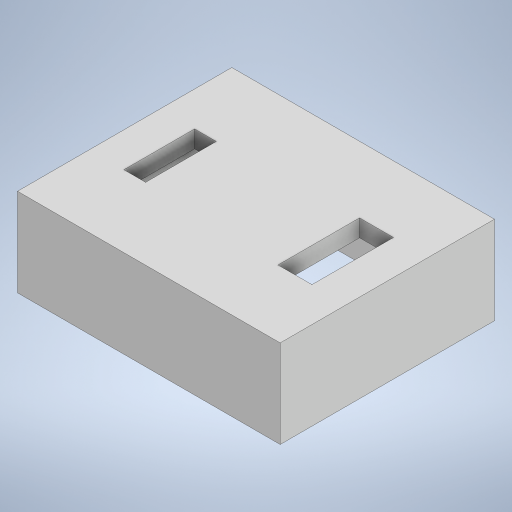
# Autodesk Inventor part: pololuCaseTop
Saved by Autodesk Inventor 2024 (Build 280153000, 153)
## iProperties
Created: 2023-08-07
Part Number: pololuCaseTop
Material: Generic
Document SubType Name: Modeling
Designer: 18179
Density: 1 g/cm^3
Appearance: Default
Author: 18179
Autodesk Inventor part; units mm, degrees
ref_plane "YZ Plane" through (0, 0, 0) normal (1, 0, 0) x (0, 1, 0)
ref_plane "XZ Plane" through (0, 0, 0) normal (0, 1, 0) x (-1, 0, 0)
ref_plane "XY Plane" through (0, 0, 0) normal (0, 0, 1) x (1, 0, 0)
sketch "Sketch1" plane through (0, 0, 0) normal (0, 1, 0) x (-1, 0, 0)
  line L0 (0, 0) -> (41.91, 0)
  line L1 (41.91, 0) -> (41.91, -33.02)
  line L2 (41.91, -33.02) -> (0, -33.02)
  line L3 (0, -33.02) -> (0, 0)
  line L4 (41.91, -16.51) -> (34.735, -16.51)
  line L5 (34.735, -16.51) -> (34.735, -10.01)
  line L6 (34.735, -10.01) -> (41.91, -10.01)
  line L7 (34.735, -10.01) -> (38.735, -10.01)
  line L8 (38.735, -10.01) -> (38.735, -23.01)
  line L9 (38.735, -23.01) -> (34.735, -23.01)
  line L10 (34.735, -23.01) -> (34.735, -10.01)
  line L11 (0, -16.51) -> (9.425, -16.51)
  line L12 (9.425, -16.51) -> (9.425, -9.01)
  line L13 (9.425, -9.01) -> (3.175, -9.01)
  line L14 (3.175, -9.01) -> (3.175, -24.01)
  line L15 (3.175, -24.01) -> (9.425, -24.01)
  line L16 (9.425, -24.01) -> (9.425, -9.01)
  point P0 (0, -9.01)
  point P1 (0, -24.01)
  point P2 (41.91, -23.01)
  point P3 (3.175, -16.51)
  point P4 (38.735, -16.51)
  dimension "d0" = 41.91
  dimension "d1" = 33.02
  dimension "d2" = 7.175
  dimension "d3" = 6.5
  dimension "d4" = 4
  dimension "d5" = 13
  dimension "d6" = 9.425
  dimension "d7" = 7.5
  dimension "d8" = 6.25
  dimension "d9" = 15
  constraints: 34 end point, 6 parallel, 6 perpendicular, 5 horizontal, 2 midpoint, 1 point on line
  measures "d0" distance of L1.end L2.end
  measures "d1" distance of L0.end L1.end
  measures "d2" distance of L4.start L4.end
  measures "d3" distance of L4.end L5.end
  measures "d4" distance of L8.end L9.end
  measures "d5" distance of L7.end L8.end
  measures "d6" distance of L11.start L11.end
  measures "d7" distance of L11.end L12.end
  measures "d8" distance of L15.end L14.end
  measures "d9" distance of L14.end L13.end
extrude "Extrusion1" add sketch "Sketch1" along normal blind 3.175 contours L0 L1 L6 L5 L10 L9 L8 L4 L2 L3 | L1 L4 L8 L6
sketch "Sketch2" plane through (0, 3.175, 0) normal (0, 1, 0) x (1, 0, 0)
  line L0 (0, 0) -> (0, 33.02) projected
  line L1 (-3.175, 9.01) -> (-9.425, 9.01) projected
  line L2 (-9.425, 9.01) -> (-9.425, 24.01) projected
  line L3 (-9.425, 24.01) -> (-3.175, 24.01) projected
  line L4 (0, 33.02) -> (-41.91, 33.02) projected
  line L5 (-41.91, 33.02) -> (-41.91, 0) projected
  line L6 (-38.735, 23.01) -> (-34.735, 23.01) projected
  line L7 (-34.735, 23.01) -> (-34.735, 10.01) projected
  line L8 (-41.91, 0) -> (0, 0) projected
  line L9 (3.175, -3.175) -> (3.175, 12.185)
  line L10 (3.175, 12.185) -> (-6.25, 12.185)
  line L11 (-6.25, 12.185) -> (-6.25, 20.835)
  line L12 (-6.25, 20.835) -> (3.175, 20.835)
  line L13 (3.175, 20.835) -> (3.175, 36.195)
  line L14 (3.175, 36.195) -> (-45.085, 36.195)
  line L15 (-45.085, 36.195) -> (-45.085, 19.835)
  line L16 (-45.085, 19.835) -> (-37.91, 19.835)
  line L17 (-37.91, 19.835) -> (-37.91, 13.185)
  line L18 (-37.91, 13.185) -> (-45.085, 13.185)
  line L19 (-45.085, 13.185) -> (-45.085, -3.175)
  line L20 (-45.085, -3.175) -> (3.175, -3.175)
  line L21 (3.175, 12.185) -> (3.175, 20.835)
  line L22 (0, 24.01) -> (0, 9.01)
  line L23 (-41.91, 10.01) -> (-41.91, 23.01)
  line L24 (-45.085, 19.835) -> (-45.085, 13.185)
  line L25 (-3.175, 24.01) -> (-3.175, 9.01) projected
  line L26 (-38.735, 10.01) -> (-38.735, 23.01) projected
  line L27 (-34.735, 10.01) -> (-38.735, 10.01) projected
  point P0 (-41.91, 19.835)
  point P1 (0, 20.835)
  point P2 (-3.175, 20.835)
  point P3 (-3.175, 12.185)
  point P4 (0, 12.185)
  point P5 (-41.91, 13.185)
  point P6 (-38.735, 13.185)
  point P7 (-38.735, 19.835)
  dimension "d12" = 3.175
  constraints: 32 end point, 2 parallel, 1 vertical, 6 other
  measures "d12" distance between parallel lines of L8 L20
extrude "Extrusion2" add sketch "Sketch2" against normal blind 16.1648 contours L0 L10 L9 L20 L19 L18 L5 L8 | L0 L12 L21 L10 | L0 L4 L5 L16 L15 L14 L13 L12 | L18 L24 L16 L5
body "Solid1"
